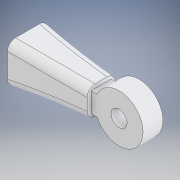
# Autodesk Inventor part: Arm2
Saved by Autodesk Inventor 2017 SP1 (Build 210196100, 196)
## iProperties
Created: 2018-02-11
Part Number: Arm2
Material: ABS Plastic
Document SubType Name: Modeling
Designer: Zach
Density: 1.06 g/cm^3
Appearance: CR White
Author: Zach
Autodesk Inventor part; units mm, degrees
ref_plane "XZ Plane" through (0, 0, 0) normal (0, 1, 0) x (-1, 0, 0)
ref_plane "XY Plane" through (0, 0, 0) normal (0, 0, 1) x (1, 0, 0)
sketch "Sketch1" plane through (0, 0, 0) normal (0, 0, 1) x (1, 0, 0)
  circle A0 centre (0, 0) radius 2
  circle A1 centre (0, 0) radius 6
  dimension "d0" = 4
  dimension "d1" = 12
  constraints: 2 centre point, 2 coincident
  measures "d0" diameter of A0
  measures "d1" diameter of A1
extrude "Extrusion1" add sketch "Sketch1" along normal blind 5
ref_plane "Work Plane1" through (-2.5, 0, 0) normal (1, 0, 0) x (0, 1, 0)
sketch "Sketch5" plane through (-2.5, 0, 0) normal (1, 0, 0) x (0, 1, 0)
  line L0 (2.5, 0) -> (-2.5, 0)
  line L1 (-2.5, 0) -> (-2.5, 5)
  line L2 (-2.5, 5) -> (2.5, 5)
  line L3 (2.5, 5) -> (2.5, 0)
  point P0 (0, 0)
  point P1 (0, 0)
  dimension "d5" = 5
  dimension "d6" = 5
  constraints: 8 end point, 2 parallel, 1 coincident, 1 horizontal, 1 midpoint, 1 perpendicular
  measures "d5" distance of L1.end L2.end
  measures "d6" distance of L0.end L1.end
extrude "Extrusion2" add sketch "Sketch5" against normal blind 6
sketch "Sketch7" plane through (-8.5, 0, 0) normal (-1, 0, 0) x (0, 0, 1)
  line L0 (0, 2.5) -> (0, -2.5) projected
  line L1 (0, -2.5) -> (5, -2.5) projected
  line L2 (5, -2.5) -> (5, 2.5) projected
  line L3 (5, 2.5) -> (0, 2.5) projected
  point P0 (0, 0)
extrude "Extrusion3" add sketch "Sketch7" along normal blind 17
sketch "Sketch8" plane through (0, 0, 5) normal (0, 0, 1) x (1, 0, 0)
  line L0 (-25.5, 5) -> (-25.5, -5)
  line L1 (-25.5, -2.5) -> (-25.5, 2.5) projected
  line L2 (-7, 3.5) -> (-7, -3.5)
  arc A0 (-25.5, 5) -> (-7, 3.5) centre (7.9832, 303.1256) ccw
  arc A1 (-7, -3.5) -> (-25.5, -5) centre (7.9832, -303.1256) ccw
  point P0 (0, 0)
  point P1 (-25.5, 0)
  point P2 (-25.5, 0)
  point P3 (-7, 0)
  dimension "d11" = 10
  dimension "d12" = 7
  dimension "d13" = 7
  dimension "d14" = 300
  dimension "d15" = 300
  constraints: 4 end point, 4 midpoint, 4 point on circle, 2 centre point, 2 vertical, 1 horizontal alignment
  measures "d11" distance of L0.start L0.end
  measures "d12" distance of L2.start L2.end
  measures "d13" distance from line of point (0, 0) L2
  measures "d14" radius of A0
  measures "d15" radius of A1
extrude "Extrusion4" add sketch "Sketch8" against normal blind 6 and the other way blind 1
sketch "Sketch9" plane through (-5.4544, 2.5, 5) normal (0, 1, 0) x (1, 0, 0)
  line L0 (-20.0456, 7.5) -> (-20.0456, -2.5) construction
  line L1 (-20.0456, -1) -> (-20.0456, 6) projected
  line L2 (-1.5456, 6) -> (-1.5456, -1)
  arc A0 (-20.0456, 7.5) -> (-1.5456, 6) centre (13.4375, 305.6256) ccw
  arc A1 (-1.5456, -1) -> (-20.0456, -2.5) centre (13.4375, -300.6256) ccw
  line L3 (-1.5456, 6) -> (-1.5456, -1) projected
  line L4 (-20.0456, 6) -> (-1.5456, 6)
  line L5 (-20.0456, -1) -> (-1.5456, -1)
  line L6 (-20.0456, 6) -> (-20.0456, 7.5)
  line L7 (-20.0456, -2.5) -> (-20.0456, -1)
  point P0 (5.4544, 5)
  point P1 (-20.0456, 2.5)
  dimension "d20" = 10
  dimension "d21" = 300
  dimension "d22" = 300
  constraints: 12 end point, 4 point on circle, 3 vertical, 2 centre point, 2 horizontal, 2 midpoint, 1 collinear
  measures "d20" distance of L0.start L0.end
  measures "d21" radius of A0
  measures "d22" radius of A1
extrude "Extrusion5" add sketch "Sketch9" along normal blind 2.5 and the other way blind 7.5 contours L5 A1 L7 | L6 A0 L4
sketch "Sketch10" plane through (-25.5, 5, -1) normal (0, 0, 1) x (1, 0, 0)
  arc A0 (0, 0) -> (18.5, -1.5) centre (33.4832, 298.1256) ccw projected
  line L0 (18.5, -1.5) -> (18.5, 0) projected
  line L1 (0, 0) -> (18.5, 0) projected
  arc A1 (18.5, -8.5) -> (0, -10) centre (33.4832, -308.1256) ccw projected
  line L2 (18.5, -10) -> (0, -10) projected
  line L3 (18.5, -10) -> (18.5, -8.5) projected
  point P0 (25.5, -5)
extrude "Extrusion6" cut sketch "Sketch10" along normal through all both and the other way through all
fillet "Fillet1" radius 2 4 edges at (-16.2955, 4.1096, 6.6096) (-16.2616, 4.1069, -1.6069) (-16.2616, -4.1069, 6.6069) (-16.2955, -4.1096, -1.6096)
sketch "Sketch11" plane through (-25.5, 0, 0) normal (-1, 0, 0) x (0, 0, 1)
  circle A0 centre (2.5, 0) radius 1.5
  line L0 (5.5125, 5) -> (-0.5125, 5) projected
  line L1 (7.5, 3.0125) -> (7.5, -3.0125) projected
  point P0 (0, 0)
  point P1 (7.5, 0)
  point P2 (2.5, 5)
  dimension "d30" = 3
  constraints: 2 midpoint, 1 centre point, 1 horizontal alignment, 1 vertical alignment
  measures "d30" diameter of A0
extrude "Extrusion7" cut sketch "Sketch11" against normal blind 10
body "Solid1"
